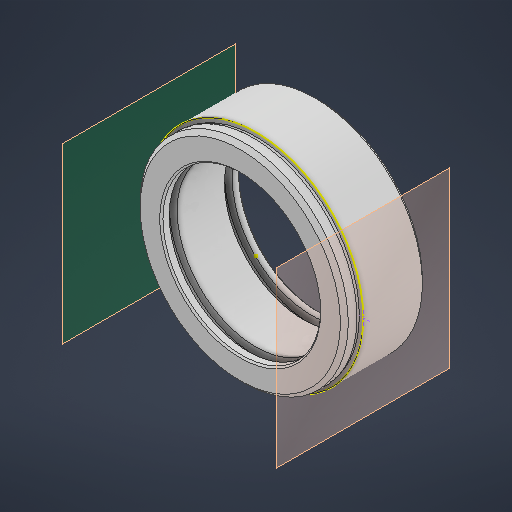
# Autodesk Inventor part: tuleja łożyska
Saved by Autodesk Inventor 2026.1 (Build 301233020, 233B)
## iProperties
Created: 2026-02-27
Part Number: tuleja łożyska
Material: Generic
Document SubType Name: Modeling
Designer: Jan
Density: 1 g/cm^3
Appearance: Default
Author: Jan
Autodesk Inventor part; units mm, degrees
ref_plane "YZ Plane" through (0, 0, 0) normal (1, 0, 0) x (0, 1, 0)
ref_plane "XZ Plane" through (0, 0, 0) normal (0, 1, 0) x (-1, 0, 0)
ref_plane "XY Plane" through (0, 0, 0) normal (0, 0, 1) x (1, 0, 0)
sketch "Sketch4" plane through (0, 0, 0) normal (0, 1, 0) x (-1, 0, 0)
  line L0 (-13.6, -3.4347) -> (-13.6, -11.4347)
  line L1 (-11, -9.4347) -> (-10, -9.4347)
  line L2 (-11, -3.4347) -> (-10, -3.4347)
  line L3 (-10, -3.4347) -> (-10, -9.4347)
  line L4 (0, 0) -> (0, -21.3586) construction
  line L5 (-10, -11.4347) -> (-13.6, -11.4347)
  line L6 (-10, -1.4347) -> (-12, -1.4347)
  line L7 (-11, -9.4347) -> (-11, -10.4347)
  line L8 (-11, -10.4347) -> (-10, -10.4347)
  line L9 (-11, -3.4347) -> (-11, -2.4347)
  line L10 (-11, -2.4347) -> (-10, -2.4347)
  line L11 (-10, -1.4347) -> (-10, -2.4347)
  line L12 (-10, -10.4347) -> (-10, -11.4347)
  line L13 (-13.2, -1.4347) -> (-12, -1.4347)
  line L14 (-13.2, -3.0347) -> (-13.2, -1.4347)
  line L15 (-13.6, -3.4347) -> (-13.1, -3.4347)
  line L16 (-13.1, -3.4347) -> (-13.1, -3.0347)
  line L17 (-13.1, -3.0347) -> (-13.2, -3.0347)
  point P0 (-10, -10.9347)
  point P1 (-11, -9.9347)
  dimension "d23" = 8
  dimension "d28" = 6
  dimension "d29" = 10
  dimension "d37" = 1
  dimension "d38" = 1
  dimension "d39" = 10
  dimension "d40" = 11
  dimension "d41" = 11
  dimension "d42" = 1
  dimension "d43" = 10
  dimension "d44" = 2
  dimension "d63" = 0.5
  dimension "d64" = 13.6
  dimension "d65" = 13.2
  constraints: 36 end point, 7 perpendicular, 4 horizontal, 4 vertical, 2 midpoint, 1 coincident, 1 parallel
  measures "d23" distance of L0.end L0.start
  measures "d28" distance of L2.end L1.end
  measures "d29" distance from line of L3 point (0, 0)
  measures "d37" distance of L1.start L7.end
  measures "d38" distance of L2.start L9.end
  measures "d39" horizontal distance of point (-10, -10.935) point (0, 0)
  measures "d40" distance from line of point (-11, -9.935) L4
  measures "d41" distance between parallel lines of L4 L9
  measures "d42" distance of L6.start L10.end
  measures "d43" distance from line of point (0, 0) L11
  measures "d44" distance of L6.start L6.end
  measures "d63" distance of L0.start L15.end
  measures "d64" distance between parallel lines of L4 L0
  measures "d65" distance from line of L14 L4.start
revolve "Revolution1" add sketch "Sketch4" angle 360 about axis through (0, 0, 0) along (0, 0, -1)
chamfer "Chamfer1" distance 0.5 angle 45 1 edges at (-13.2, 0, -1.4347)
sketch "Sketch5" plane through (0, 0, -3.4347) normal (0, 0, 1) x (1, 0, 0)
  circle A0 centre (0, 0) radius 13.6 projected
  point P0 (13.6, 0)
  point P1 (-13.6, 0)
  constraints: 2 point on circle
ref_plane "Work Plane1" through (13.6, 0, -3.4347) normal (1, 0, 0) x (0, 1, 0)
ref_plane "Work Plane2" through (-13.6, 0, -3.4347) normal (-1, 0, 0) x (0, -1, 0)
chamfer "Chamfer2" distance 0.5 angle 45 1 edges at (-13.6, 0, -11.4347)
chamfer "Chamfer3" distance 0.2 angle 45 1 edges at (-10, 0, -1.4347)
chamfer "Chamfer4" distance 0.2 angle 45 1 edges at (-10, 0, -11.4347)
body "Solid2"
